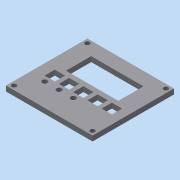
# Autodesk Inventor part: Schiled
Saved by Autodesk Inventor 2018 (Build 220112000, 112)
## iProperties
Created: 2020-10-03
Part Number: Schiled
Material: Generisch
Document SubType Name: Modeling
Designer: marce
Density: 1 g/cm^3
Appearance: Vorgabe
Author: marce
Autodesk Inventor part; units mm, degrees
ref_plane "YZ Plane" through (0, 0, 0) normal (1, 0, 0) x (0, 1, 0)
ref_plane "XZ Plane" through (0, 0, 0) normal (0, 1, 0) x (-1, 0, 0)
ref_plane "XY Plane" through (0, 0, 0) normal (0, 0, 1) x (1, 0, 0)
sketch "Skizze1" plane through (0, 0, 0) normal (0, 0, 1) x (1, 0, 0)
  line L0 (0, 0) -> (85, 0)
  line L1 (85, 0) -> (85, 80)
  line L2 (85, 80) -> (0, 80)
  line L3 (0, 80) -> (0, 0)
  dimension "d0" = 85
  dimension "d1" = 80
  constraints: 8 end point, 2 parallel, 1 horizontal, 1 perpendicular
  measures "d0" distance of L2.end L1.end
  measures "d1" distance of L1.end L0.end
extrude "Extrusion1" add sketch "Skizze1" along normal blind 5
sketch "Skizze3" plane through (0, 0, 5) normal (0, 0, 1) x (1, 0, 0)
  line L0 (7.5, 71) -> (77.5, 71)
  line L1 (77.5, 71) -> (77.5, 9)
  line L2 (77.5, 9) -> (7.5, 9)
  line L3 (7.5, 9) -> (7.5, 71)
  line L4 (85, 80) -> (0, 80) projected
  line L5 (85, 0) -> (85, 80) projected
  line L6 (16.85, 66.85) -> (68.15, 66.85)
  line L7 (68.15, 66.85) -> (68.15, 42.15)
  line L8 (68.15, 42.15) -> (16.85, 42.15)
  line L9 (16.85, 42.15) -> (16.85, 66.85)
  line L10 (10.5, 37.5) -> (20.5, 37.5)
  line L11 (20.5, 37.5) -> (20.5, 27.5)
  line L12 (20.5, 27.5) -> (10.5, 27.5)
  line L13 (10.5, 27.5) -> (10.5, 37.5)
  line L14 (15.5, 37.5) -> (15.5, 27.5)
  line L15 (10.5, 32.5) -> (20.5, 32.5)
  line L16 (24.5, 37.5) -> (34.5, 37.5)
  line L17 (34.5, 37.5) -> (34.5, 27.5)
  line L18 (34.5, 27.5) -> (24.5, 27.5)
  line L19 (24.5, 27.5) -> (24.5, 37.5)
  line L20 (38.5, 37.5) -> (48.5, 37.5)
  line L21 (48.5, 37.5) -> (48.5, 27.5)
  line L22 (48.5, 27.5) -> (38.5, 27.5)
  line L23 (38.5, 27.5) -> (38.5, 37.5)
  line L24 (52.5, 37.5) -> (62.5, 37.5)
  line L25 (62.5, 37.5) -> (62.5, 27.5)
  line L26 (62.5, 27.5) -> (52.5, 27.5)
  line L27 (52.5, 27.5) -> (52.5, 37.5)
  line L28 (66.5, 37.5) -> (76.5, 37.5)
  line L29 (76.5, 37.5) -> (76.5, 27.5)
  line L30 (76.5, 27.5) -> (66.5, 27.5)
  line L31 (66.5, 27.5) -> (66.5, 37.5)
  point P0 (0, 0)
  point P1 (77.5, 40)
  point P2 (85, 40)
  point P3 (42.5, 71)
  point P4 (42.5, 80)
  point P5 (42.5, 66.85)
  dimension "d9" = 70
  dimension "d10" = 62
  dimension "d12" = 51.3
  dimension "d13" = 24.7
  dimension "d14" = 4.15
  dimension "d15" = 10
  dimension "d16" = 10
  dimension "d21" = 8
  dimension "d22" = 23.5
  dimension "d23" = 14
  dimension "d24" = 14
  dimension "d25" = 14
  dimension "d26" = 14
  constraints: 60 end point, 14 parallel, 9 midpoint, 7 equal length, 7 horizontal, 7 perpendicular, 3 point on line, 2 collinear, 2 vertical alignment, 1 horizontal alignment
  measures "d9" distance of L1.end L2.end
  measures "d10" distance of L0.end L1.end
  measures "d12" distance of L7.end L8.end
  measures "d13" distance of L6.end L7.end
  measures "d14" distance between parallel lines of L0 L6
  measures "d15" distance of L11.end L12.end
  measures "d16" distance of L10.end L11.end
  measures "d21" distance between parallel lines of L14 L3
  measures "d22" distance between parallel lines of L2 L15
  measures "d23" distance between parallel lines of L19 L13
  measures "d24" distance between parallel lines of L23 L19
  measures "d25" distance between parallel lines of L23 L27
  measures "d26" distance between parallel lines of L27 L31
extrude "Extrusion3" cut sketch "Skizze3" against normal through all contours L6 L7 L8 L9 | L10 L14 L15 L13 | L10 L11 L15 L14 | L15 L14 L12 L13 | L15 L11 L12 L14 | L16 L17 L18 L19 | L20 L21 L22 L23 | L24 L25 L26 L27 | L28 L29 L30 L31
sketch "Skizze5" plane through (0, 0, 0) normal (0, 0, -1) x (-1, 0, 0)
  line L0 (-20.5, 27.5) -> (-20.5, 37.5) projected
  line L1 (-20.5, 37.5) -> (-10.5, 37.5) projected
  line L2 (-10.5, 37.5) -> (-10.5, 27.5) projected
  line L3 (-10.5, 27.5) -> (-20.5, 27.5) projected
  line L4 (-66.5, 37.5) -> (-66.5, 27.5) projected
  line L5 (-66.5, 27.5) -> (-76.5, 27.5) projected
  line L6 (-76.5, 27.5) -> (-76.5, 37.5) projected
  line L7 (-76.5, 37.5) -> (-66.5, 37.5) projected
  line L8 (-38.5, 37.5) -> (-38.5, 27.5) projected
  line L9 (-38.5, 27.5) -> (-48.5, 27.5) projected
  line L10 (-48.5, 27.5) -> (-48.5, 37.5) projected
  line L11 (-48.5, 37.5) -> (-38.5, 37.5) projected
  line L12 (-24.5, 37.5) -> (-24.5, 27.5) projected
  line L13 (-24.5, 27.5) -> (-34.5, 27.5) projected
  line L14 (-34.5, 27.5) -> (-34.5, 37.5) projected
  line L15 (-34.5, 37.5) -> (-24.5, 37.5) projected
  line L16 (-52.5, 37.5) -> (-52.5, 27.5) projected
  line L17 (-52.5, 27.5) -> (-62.5, 27.5) projected
  line L18 (-62.5, 27.5) -> (-62.5, 37.5) projected
  line L19 (-62.5, 37.5) -> (-52.5, 37.5) projected
  line L20 (-16.85, 66.85) -> (-16.85, 42.15) projected
  line L21 (-16.85, 42.15) -> (-68.15, 42.15) projected
  line L22 (-68.15, 42.15) -> (-68.15, 66.85) projected
  line L23 (-68.15, 66.85) -> (-16.85, 66.85) projected
  line L24 (0, 0) -> (-85, 0) projected
  line L25 (0, 80) -> (0, 0) projected
  line L26 (-85, 80) -> (0, 80) projected
  line L27 (-85, 0) -> (-85, 80) projected
  line L28 (-4, 76) -> (-4, 4)
  line L29 (-4, 4) -> (-81, 4)
  line L30 (-81, 4) -> (-81, 76)
  line L31 (-81, 76) -> (-4, 76)
  line L32 (-85, 80) -> (0, 80) projected
  dimension "d39" = 4
  constraints: 8 end point, 3 other
  measures "d39" distance between parallel lines of L32 L31
hole "Bohrung2" at (4, 76, 0) at (4, 4, 0) at (81, 4, 0) at (81, 76, 0) direction (0, 0, 1) diameter 4.5 end through all
sketch "Skizze6" plane through (0, 0, 0) normal (0, 0, -1) x (-1, 0, 0)
  circle A0 centre (-15.65, 22.5) radius 2.45 projected
  circle A1 centre (-29.65, 22.5) radius 2.45 projected
  circle A2 centre (-43.65, 22.5) radius 2.45 projected
  point P0 (0, 0)
hole "Bohrung3" at (43.65, 22.5, 0) at (29.65, 22.5, 0) at (15.65, 22.5, 0) direction (0, 0, 1) diameter 5 end through all
fillet "Rundung2" radius 2 4 edges at (85, 0, 2.5) (0, 0, 2.5) (0, 80, 2.5) (85, 80, 2.5)
fillet "Rundung1" radius 2 20 edges at (10.5, 37.5, 2.5) (10.5, 27.5, 2.5) (20.5, 27.5, 2.5) (20.5, 37.5, 2.5) (24.5, 37.5, 2.5) (24.5, 27.5, 2.5) (34.5, 27.5, 2.5) (34.5, 37.5, 2.5) (38.5, 37.5, 2.5) (48.5, 37.5, 2.5) (52.5, 37.5, 2.5) (62.5, 37.5, 2.5) (66.5, 37.5, 2.5) (76.5, 37.5, 2.5) (76.5, 27.5, 2.5) (66.5, 27.5, 2.5) (62.5, 27.5, 2.5) (52.5, 27.5, 2.5) (48.5, 27.5, 2.5) (38.5, 27.5, 2.5)
